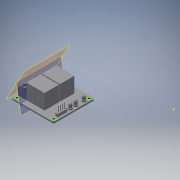
# Autodesk Inventor part: relay_module
Saved by Autodesk Inventor 2016 (Build 200138000, 138)
## iProperties
Created: 2015-11-16
Part Number: relay_module
Material: Generic
Document SubType Name: Modeling
Designer: Jufo
Density: 1 g/cm^3
Appearance: Default
Author: Jufo
Autodesk Inventor part; units mm, degrees
ref_plane "YZ Plane" through (0, 0, 0) normal (1, 0, 0) x (0, 1, 0)
ref_plane "XZ Plane" through (0, 0, 0) normal (0, 1, 0) x (-1, 0, 0)
ref_plane "XY Plane" through (0, 0, 0) normal (0, 0, 1) x (1, 0, 0)
sketch "Sketch1" plane through (0, 0, 0) normal (0, 1, 0) x (-1, 0, 0)
  line L0 (94.2568, 73.4599) -> (94.2568, 30.8599)
  line L1 (94.2568, 30.8599) -> (50.7568, 30.8599)
  line L2 (50.7568, 30.8599) -> (50.7568, 73.4599)
  line L3 (50.7568, 73.4599) -> (94.2568, 73.4599)
  point P0 (0, 0)
  dimension "d0" = 42.6
  dimension "d1" = 43.5
  constraints: 8 end point, 2 perpendicular, 2 vertical
  measures "d0" distance of L0.start L0.end
  measures "d1" distance of L0.end L1.end
extrude "Extrusion1" add sketch "Sketch1" along normal blind 1.6
sketch "Sketch2" plane through (0, 1.6, 0) normal (0, 1, 0) x (1, 0, 0)
  circle A0 centre (-53.6568, -70.5599) radius 1.5
  circle A1 centre (-53.6568, -33.9599) radius 1.5
  line L0 (-94.2568, -73.4599) -> (-50.7568, -73.4599) projected
  line L1 (-50.7568, -73.4599) -> (-50.7568, -30.8599) projected
  circle A2 centre (-91.6568, -33.9599) radius 1.5
  circle A3 centre (-91.6568, -70.5599) radius 1.5
  line L2 (-94.2568, -30.8599) -> (-94.2568, -73.4599) projected
  point P0 (0, 0)
  dimension "d4" = 3
  dimension "d5" = 3
  dimension "d6" = 36.6
  dimension "d7" = 2.9
  dimension "d8" = 2.9
  dimension "d9" = 2.9
  dimension "d10" = 3
  dimension "d11" = 38
  dimension "d12" = 3
  dimension "d13" = 38
  dimension "d14" = 2.6
  constraints: 4 centre point
  measures "d4" diameter of A0
  measures "d5" diameter of A1
  measures "d6" distance of A1.centre A0.centre
  measures "d7" distance from line of L0 A0.centre
  measures "d8" distance from line of L1 A0.centre
  measures "d9" distance from line of L1 A1.centre
  measures "d10" diameter of A2
  measures "d11" distance of A1.centre A2.centre
  measures "d12" diameter of A3
  measures "d13" distance of A0.centre A3.centre
  measures "d14" distance from line of L2 A3.centre
extrude "Extrusion2" cut sketch "Sketch2" against normal blind 1.6
sketch "Sketch3" plane through (0, 1.6, 0) normal (0, 1, 0) x (1, 0, 0)
  line L0 (-65.7568, -67.8599) -> (-65.7568, -52.8599)
  line L1 (-65.7568, -51.8599) -> (-65.7568, -36.8599)
  line L2 (-50.7568, -73.4599) -> (-50.7568, -30.8599) projected
  line L3 (-65.7568, -67.8599) -> (-84.5568, -67.8599)
  line L4 (-84.5568, -67.8599) -> (-84.5568, -52.8599)
  line L5 (-84.5568, -52.8599) -> (-65.7568, -52.8599)
  line L6 (-65.7568, -51.8599) -> (-84.5568, -51.8599)
  line L7 (-84.5568, -51.8599) -> (-84.5568, -36.8599)
  line L8 (-84.5568, -36.8599) -> (-65.7568, -36.8599)
  line L9 (-94.2568, -73.4599) -> (-50.7568, -73.4599) projected
  point P0 (0, 0)
  dimension "d17" = 15
  dimension "d18" = 15
  dimension "d19" = 15
  dimension "d20" = 15
  dimension "d21" = 18.8
  dimension "d22" = 5.6
  dimension "d23" = 1
  constraints: 16 end point, 3 perpendicular, 2 point on line, 2 vertical, 1 horizontal, 1 parallel
  measures "d17" distance between parallel lines of L2 L1
  measures "d18" distance between parallel lines of L2 L0
  measures "d19" distance of L0.start L0.end
  measures "d20" distance of L1.start L1.end
  measures "d21" distance of L0.start L3.end
  measures "d22" distance between parallel lines of L9 L3
  measures "d23" distance between parallel lines of L6 L5
sketch "Sketch4" plane through (0, 1.6, 0) normal (0, 1, 0) x (1, 0, 0)
  line L0 (-55.2568, -67.1599) -> (-55.2568, -57.1599)
  line L1 (-55.2568, -57.1599) -> (-52.7568, -57.1599)
  line L2 (-52.7568, -57.1599) -> (-52.7568, -67.1599)
  line L3 (-52.7568, -67.1599) -> (-55.2568, -67.1599)
  line L4 (-50.7568, -73.4599) -> (-50.7568, -30.8599) projected
  line L5 (-94.2568, -73.4599) -> (-50.7568, -73.4599) projected
  point P0 (0, 0)
  dimension "d26" = 10
  dimension "d27" = 2
  dimension "d28" = 2.5
  dimension "d29" = 6.3
  constraints: 8 end point, 3 perpendicular, 1 vertical
  measures "d26" distance of L0.start L0.end
  measures "d27" distance between parallel lines of L4 L2
  measures "d28" distance of L0.end L1.end
  measures "d29" distance between parallel lines of L5 L3
extrude "Extrusion4" add sketch "Sketch4" along normal blind 3
sketch "Sketch5" plane through (0, 4.6, 0) normal (0, 1, 0) x (1, 0, 0)
  circle A0 centre (-54.0568, -65.3099) radius 0.3
  circle A1 centre (-54.0568, -63.2099) radius 0.3
  circle A2 centre (-54.0568, -61.1099) radius 0.3
  circle A3 centre (-54.0568, -59.0099) radius 0.3
  line L0 (-55.2568, -67.1599) -> (-52.7568, -67.1599) projected
  line L1 (-52.7568, -67.1599) -> (-52.7568, -57.1599) projected
  point P0 (0, 0)
  dimension "d32" = 0.6
  dimension "d33" = 0.6
  dimension "d34" = 0.6
  dimension "d35" = 0.6
  dimension "d36" = 1.85
  dimension "d37" = 1.3
  dimension "d38" = 2.1
  dimension "d39" = 2.1
  dimension "d40" = 2.1
  dimension "d41" = 1.3
  constraints: 4 centre point
  measures "d32" diameter of A0
  measures "d33" diameter of A1
  measures "d34" diameter of A2
  measures "d35" diameter of A3
  measures "d36" distance from line of A0.centre L0
  measures "d37" distance from line of L1 A0.centre
  measures "d38" distance of A1.centre A0.centre
  measures "d39" distance of A2.centre A1.centre
  measures "d40" distance of A2.centre A3.centre
  measures "d41" distance from line of L1 A1.centre
extrude "Extrusion5" add sketch "Sketch5" along normal blind 5.8
sketch "Sketch6" plane through (0, 1.6, 0) normal (0, 1, 0) x (1, 0, 0)
  circle A0 centre (-54.0568, -38.8599) radius 2
  circle A1 centre (-54.0568, -47.2599) radius 2
  circle A2 centre (-54.0568, -52.7599) radius 2
  circle A3 centre (-53.6568, -33.9599) radius 1.5 projected
  line L0 (-50.7568, -30.8599) -> (-94.2568, -30.8599) projected
  line L1 (-50.7568, -30.8599) -> (-50.7568, -73.4599) projected
  point P0 (0, 0)
  dimension "d44" = 4
  dimension "d45" = 4
  dimension "d46" = 4
  dimension "d48" = 8
  dimension "d49" = 8.4
  dimension "d50" = 5.5
  dimension "d51" = 3.3
  constraints: 3 centre point
  measures "d44" diameter of A0
  measures "d45" diameter of A1
  measures "d46" diameter of A2
  measures "d48" distance from line of L0 A0.centre
  measures "d49" distance of A1.centre A0.centre
  measures "d50" distance of A1.centre A2.centre
  measures "d51" distance from line of L1 A0.centre
extrude "Extrusion6" add sketch "Sketch6" along normal blind 1.2 contours A0 | A1 | A2
sketch "Sketch7" plane through (-54.0568, 2.8, 52.7599) normal (0, 1, 0) x (1, 0, 0)
  circle A0 centre (0, 0) radius 2 projected
  circle A1 centre (0, 0) radius 1.5
  point P0 (54.0568, 52.7599)
  dimension "d54" = 3
  constraints: 1 centre point, 1 coincident
  measures "d54" diameter of A1
sketch "Sketch8" plane through (-54.0568, 2.8, 47.2599) normal (0, 1, 0) x (1, 0, 0)
  circle A0 centre (0, 0) radius 2 projected
  circle A1 centre (0, 0) radius 1.5
  point P0 (54.0568, 47.2599)
  dimension "d55" = 3
  constraints: 1 centre point, 1 coincident
  measures "d55" diameter of A1
sketch "Sketch9" plane through (-54.0568, 2.8, 38.8599) normal (0, 1, 0) x (1, 0, 0)
  circle A0 centre (0, 0) radius 2 projected
  circle A1 centre (0, 0) radius 1.5
  point P0 (54.0568, 38.8599)
  dimension "d56" = 3
  constraints: 1 centre point, 1 coincident
  measures "d56" diameter of A1
extrude "Extrusion7" add sketch "Sketch7" along normal blind 4.3 contours A1
extrude "Extrusion8" add sketch "Sketch8" along normal blind 4.3 contours A1
extrude "Extrusion9" add sketch "Sketch9" along normal blind 4.3 contours A1
fillet "Fillet1" radius 1.5 3 edges at (-55.5568, 7.1, 52.7599) (-55.5568, 7.1, 47.2599) (-55.5568, 7.1, 38.8599)
sketch "Sketch10" plane through (0, 1.6, 0) normal (0, 1, 0) x (1, 0, 0)
  line L0 (-85.2568, -36.9599) -> (-85.2568, -51.9599)
  line L1 (-85.2568, -51.9599) -> (-93.2568, -51.9599)
  line L2 (-93.2568, -51.9599) -> (-93.2568, -36.9599)
  line L3 (-93.2568, -36.9599) -> (-85.2568, -36.9599)
  line L4 (-93.2568, -52.9599) -> (-85.2568, -52.9599)
  line L5 (-85.2568, -52.9599) -> (-85.2568, -67.9599)
  line L6 (-85.2568, -67.9599) -> (-93.2568, -67.9599)
  line L7 (-93.2568, -67.9599) -> (-93.2568, -52.9599)
  line L8 (-84.5568, -36.8599) -> (-84.5568, -51.8599) projected
  line L9 (-50.7568, -30.8599) -> (-94.2568, -30.8599) projected
  point P0 (0, 0)
  dimension "d64" = 8
  dimension "d65" = 0.7
  dimension "d66" = 6.1
  dimension "d67" = 15
  dimension "d68" = 15
  dimension "d69" = 1
  constraints: 16 end point, 4 perpendicular, 4 point on line, 2 vertical, 1 parallel
  measures "d64" distance of L2.end L0.start
  measures "d65" distance between parallel lines of L0 L8
  measures "d66" distance between parallel lines of L9 L3
  measures "d67" distance of L1.end L2.end
  measures "d68" distance of L6.end L4.start
  measures "d69" distance between parallel lines of L1 L4
extrude "Extrusion10" add sketch "Sketch10" along normal blind 6
sketch "Sketch11" plane through (-93.2568, 1.6, 36.9599) normal (-1, 0, 0) x (0, 0, 1)
  line L0 (0.4, 0.8) -> (0.4, 5.8)
  line L1 (0.4, 5.8) -> (4.7, 5.8)
  line L2 (4.7, 5.8) -> (4.7, 0.8)
  line L3 (4.7, 0.8) -> (0.4, 0.8)
  line L4 (15, 0) -> (0, 0) projected
  line L5 (5.3, 5.8) -> (9.6, 5.8)
  line L6 (9.6, 5.8) -> (9.6, 0.8)
  line L7 (9.6, 0.8) -> (5.3, 0.8)
  line L8 (5.3, 0.8) -> (5.3, 5.8)
  line L9 (10.2, 5.8) -> (14.5, 5.8)
  line L10 (14.5, 5.8) -> (14.5, 0.8)
  line L11 (14.5, 0.8) -> (10.2, 0.8)
  line L12 (10.2, 0.8) -> (10.2, 5.8)
  line L13 (0, 0) -> (0, 6) projected
  point P0 (-36.9599, -1.6)
  dimension "d72" = 4.3
  dimension "d73" = 5
  dimension "d74" = 0.8
  dimension "d75" = 4.3
  dimension "d76" = 4.3
  dimension "d77" = 5
  dimension "d78" = 0.6
  dimension "d79" = 0.6
  dimension "d80" = 0.4
  constraints: 24 end point, 5 perpendicular, 4 parallel, 2 horizontal, 1 point on line, 1 vertical
  measures "d72" distance of L2.end L0.start
  measures "d73" distance of L1.end L2.end
  measures "d74" distance between parallel lines of L4 L3
  measures "d75" distance of L6.end L7.end
  measures "d76" distance of L10.end L11.end
  measures "d77" distance of L9.end L10.end
  measures "d78" distance between parallel lines of L2 L8
  measures "d79" distance between parallel lines of L6 L12
  measures "d80" distance between parallel lines of L13 L0
extrude "Extrusion11" cut sketch "Sketch11" against normal blind 1
sketch "Sketch12" plane through (0, 7.6, 0) normal (0, 1, 0) x (1, 0, 0)
  line L0 (-86.0568, -36.9599) -> (-91.0568, -36.9599)
  line L1 (-92.2568, -47.1599) -> (-92.2568, -51.4599) projected
  line L2 (-92.2568, -51.9599) -> (-86.0568, -51.9599)
  line L3 (-86.0568, -51.9599) -> (-86.0568, -36.9599)
  line L4 (-85.2568, -36.9599) -> (-93.2568, -36.9599) projected
  line L5 (-93.2568, -51.9599) -> (-85.2568, -51.9599) projected
  line L6 (-84.5568, -36.8599) -> (-84.5568, -51.8599) projected
  line L7 (-91.0568, -36.9599) -> (-91.0568, -51.9599)
  line L8 (-86.0568, -36.9599) -> (-91.0568, -36.9599)
  line L9 (-86.0568, -51.9599) -> (-91.0568, -51.9599)
  point P0 (0, 0)
  dimension "d83" = 0
  dimension "d84" = 0
  dimension "d85" = 1.5
  dimension "d86" = 5
  constraints: 12 end point, 3 horizontal, 2 perpendicular, 2 point on line
  measures "d83" distance between parallel lines of L4 L0
  measures "d84" distance between parallel lines of L5 L2
  measures "d85" distance between parallel lines of L6 L3
  measures "d86" distance of L0.start L0.end
extrude "Extrusion12" add sketch "Sketch12" along normal blind 4
ref_plane "Work Plane2" through (-91.0568, 11.6, 36.9599) normal (0.8762, -0.4819, 0) x (0, 0, 1)
sketch "Sketch13" plane through (-91.0568, 11.6, 36.9599) normal (0.8762, -0.4819, 0) x (0, 0, 1)
  line L0 (0, 0) -> (0, 4.5651)
  line L1 (0, 5.967) -> (0, 0.7097) projected
  line L2 (0, 4.5651) -> (15, 4.5651)
  line L3 (0, 4.5651) -> (15, 4.5651) projected
  line L4 (15, 4.5651) -> (15, 0)
  line L5 (15, 0) -> (0, 0)
  line L6 (0, 0) -> (15, 0) projected
  point P0 (-36.9599, -33.7179)
  constraints: 8 end point, 3 collinear, 1 perpendicular
extrude "Extrusion13" add sketch "Sketch13" along normal blind 2
ref_plane "Work Plane3" through (-86.0568, 11.6, 51.9599) normal (-0.9806, -0.1961, 0) x (0, 0, -1)
sketch "Sketch14" plane through (-86.0568, 11.6, 51.9599) normal (-0.9806, -0.1961, 0) x (0, 0, -1)
  line L0 (15, 0) -> (15, 4.0792)
  line L1 (15, 4.0792) -> (0, 4.0792)
  line L2 (0, 4.0792) -> (0, 0)
  line L3 (0, 0) -> (15, 0)
  line L4 (0, 0) -> (15, 0) projected
  point P0 (51.9599, 28.2519)
  constraints: 8 end point, 1 collinear, 1 horizontal, 1 perpendicular, 1 vertical
extrude "Extrusion14" add sketch "Sketch14" along normal blind 2
sketch "Sketch15" plane through (0, 11.6, 0) normal (0, 1, 0) x (1, 0, 0)
  circle A0 centre (-88.5568, -39.4599) radius 1.8
  circle A1 centre (-88.5568, -44.4599) radius 1.8
  circle A2 centre (-88.5568, -49.4599) radius 1.8
  line L0 (-86.0568, -36.9599) -> (-91.0568, -36.9599) projected
  line L1 (-91.0568, -51.9599) -> (-86.0568, -51.9599) projected
  point P0 (0, 0)
  dimension "d93" = 3.6
  dimension "d94" = 3.6
  dimension "d95" = 3.6
  dimension "d96" = 2.5
  dimension "d97" = 5
  dimension "d98" = 5
  constraints: 3 centre point
  measures "d93" diameter of A0
  measures "d94" diameter of A1
  measures "d95" diameter of A2
  measures "d96" distance from line of A0.centre L0
  measures "d97" distance of A0.centre A1.centre
  measures "d98" distance of A1.centre A2.centre
extrude "Extrusion15" cut sketch "Sketch15" against normal blind 2
sketch "Sketch16" plane through (0, 7.6, 0) normal (0, 1, 0) x (1, 0, 0)
  line L0 (-85.2568, -52.9599) -> (-86.0568, -52.9599)
  line L1 (-85.2568, -52.9599) -> (-93.2568, -52.9599) projected
  line L2 (-86.0568, -51.9599) -> (-86.0568, -36.9599) projected
  line L3 (-86.0568, -52.9599) -> (-91.0568, -52.9599)
  line L4 (-91.0568, -52.9599) -> (-91.0568, -67.9599)
  line L5 (-93.2568, -67.9599) -> (-85.2568, -67.9599) projected
  line L6 (-86.0568, -52.9599) -> (-86.0568, -67.9599)
  line L7 (-91.0568, -67.9599) -> (-86.0568, -67.9599)
  point P0 (0, 0)
  dimension "d102" = 5
  constraints: 10 end point, 4 point on line, 2 perpendicular, 1 collinear, 1 parallel
  measures "d102" distance of L0.end L3.end
extrude "Extrusion16" add sketch "Sketch16" along normal blind 4
sketch "Sketch17" plane through (-91.0568, 11.6, 36.9599) normal (0.8762, -0.4819, 0) x (0, 0, 1)
  line L0 (16, 0) -> (16, 4.5662)
  line L1 (16, 4.5662) -> (31, 4.5662)
  line L2 (31, 5.967) -> (31, 0.7097) projected
  line L3 (31, 4.5662) -> (31, 0)
  line L4 (31, 1.0953) -> (31, -2.4096) projected
  line L5 (31, 0) -> (16, 0)
  line L6 (16, 0) -> (31, 0) projected
  point P0 (-36.9599, -33.7179)
  constraints: 8 end point, 2 point on line, 1 collinear, 1 perpendicular, 1 vertical
extrude "Extrusion17" add sketch "Sketch17" along normal blind 4
sketch "Sketch18" plane through (-86.0568, 11.6, 51.9599) normal (-0.9806, -0.1961, 0) x (0, 0, -1)
  line L0 (-1, 4.0792) -> (-1, 0)
  line L1 (-1, 0) -> (-16, 0)
  line L2 (-16, 0) -> (-1, 0) projected
  line L3 (-16, 0) -> (-16, 4.0792)
  line L4 (-16, 3.9223) -> (-16, 0) projected
  line L5 (-16, 4.0792) -> (-1, 4.0792)
  line L6 (-16, 4.0792) -> (-1, 4.0792) projected
  point P0 (51.9599, 28.2519)
  constraints: 8 end point, 3 collinear, 1 vertical
extrude "Extrusion18" add sketch "Sketch18" along normal blind 4
sketch "Sketch19" plane through (0, 11.6, 0) normal (0, 1, 0) x (1, 0, 0)
  circle A0 centre (-88.5568, -55.4599) radius 1.8
  circle A1 centre (-88.5568, -60.4599) radius 1.8
  circle A2 centre (-88.5568, -65.4599) radius 1.8
  line L0 (-86.0568, -52.9599) -> (-91.0568, -52.9599) projected
  line L1 (-91.0568, -67.9599) -> (-86.0568, -67.9599) projected
  line L2 (-91.0568, -52.9599) -> (-91.0568, -67.9599) projected
  point P0 (0, 0)
  dimension "d109" = 3.6
  dimension "d110" = 3.6
  dimension "d111" = 3.6
  dimension "d112" = 2.5
  dimension "d113" = 1.4
  dimension "d115" = 1.4
  dimension "d116" = 2.5
  dimension "d117" = 2.5
  dimension "d118" = 2.5
  constraints: 3 centre point
  measures "d109" diameter of A0
  measures "d110" diameter of A1
  measures "d111" diameter of A2
  measures "d112" distance from line of L0 A0.centre
  measures "d116" distance from line of A2.centre L2
  measures "d117" distance from line of L2 A1.centre
  measures "d118" distance from line of L2 A0.centre
extrude "Extrusion19" cut sketch "Sketch19" against normal blind 2
sketch "Sketch20" plane through (-93.2568, 1.6, 52.9599) normal (-1, 0, 0) x (0, 0, 1)
  line L0 (0.4, 5.2955) -> (4.7, 5.2955)
  line L1 (4.7, 5.2955) -> (4.7, 0.2955)
  line L2 (4.7, 0.2955) -> (0.4, 0.2955)
  line L3 (0.4, 0.2955) -> (0.4, 5.2955)
  line L4 (5.3, 5.2955) -> (9.6, 5.2955)
  line L5 (9.6, 5.2955) -> (9.6, 0.2955)
  line L6 (9.6, 0.2955) -> (5.3, 0.2955)
  line L7 (5.3, 0.2955) -> (5.3, 5.2955)
  line L8 (10.2, 5.2955) -> (14.5, 5.2955)
  line L9 (14.5, 5.2955) -> (14.5, 0.2955)
  line L10 (14.5, 0.2955) -> (10.2, 0.2955)
  line L11 (10.2, 0.2955) -> (10.2, 5.2955)
  line L12 (0, 0) -> (0, 5.9988) projected
  point P0 (-52.9599, -1.6)
  dimension "d121" = 4.3
  dimension "d122" = 5
  dimension "d123" = 4.3
  dimension "d124" = 5
  dimension "d125" = 4.3
  dimension "d126" = 5
  dimension "d127" = 0.4
  dimension "d128" = 0.6
  dimension "d129" = 0.6
  constraints: 24 end point, 6 parallel, 3 horizontal, 3 perpendicular, 2 point on line
  measures "d121" distance of L1.end L2.end
  measures "d122" distance of L0.end L1.end
  measures "d123" distance of L5.end L6.end
  measures "d124" distance of L4.end L5.end
  measures "d125" distance of L9.end L10.end
  measures "d126" distance of L8.end L9.end
  measures "d127" distance between parallel lines of L12 L3
  measures "d128" distance between parallel lines of L7 L1
  measures "d129" distance between parallel lines of L5 L11
extrude "Extrusion20" cut sketch "Sketch20" against normal blind 1
extrude "Extrusion21" add sketch "Sketch3" along normal blind 15.7
chamfer "Chamfer1" distance 1 angle 45 4 edges at (-94.2568, 0.8, 30.8599) (-50.7568, 0.8, 30.8599) (-94.2568, 0.8, 73.4599) (-50.7568, 0.8, 73.4599)
fillet "Fillet2" radius 0.2 3 edges at (-56.0568, 2.8, 52.7599) (-56.0568, 2.8, 47.2599) (-56.0568, 2.8, 38.8599)
sketch "Sketch21" plane through (0, 1.6, 0) normal (0, 1, 0) x (1, 0, 0)
  circle A0 centre (-53.6568, -70.5599) radius 1.5 projected
  circle A1 centre (-53.6568, -70.5599) radius 1.5
  circle A2 centre (-91.6568, -70.5599) radius 1.5 projected
  circle A3 centre (-91.6568, -70.5599) radius 1.5
  circle A4 centre (-53.6568, -33.9599) radius 1.5 projected
  circle A5 centre (-53.6568, -33.9599) radius 1.5
  circle A6 centre (-91.6568, -33.9599) radius 1.5 projected
  circle A7 centre (-91.6568, -33.9599) radius 1.5
  point P0 (0, 0)
  constraints: 4 centre point, 4 coincident
equation "\"d41\" = d37"
equation "\"d117\" = d116"
equation "\"d118\" = d116"
body "Solid1"
